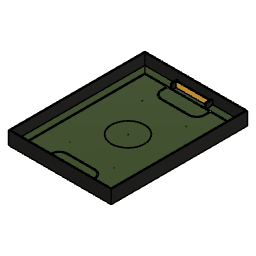
Game-field (Autodesk Fusion 360 design; units mm, degrees)
Autodesk Fusion 360 part; units mm, degrees
sketch "スケッチ1" plane through (0, 0, 0) normal (0, 1, 0) x (1, 0, 0)
  line L0 (-910, -1215) -> (910, -1215)
  line L1 (910, -1215) -> (910, 1215)
  line L2 (910, 1215) -> (-910, 1215)
  line L3 (-910, 1215) -> (-910, -1215)
  line L4 (930, 1235) -> (-930, 1235)
  line L5 (-930, 1235) -> (-930, -1235)
  line L6 (-930, -1235) -> (930, -1235)
  line L7 (930, -1235) -> (930, 1235)
extrude "押し出し1" add sketch "スケッチ1" along normal blind 20 contours L0 L1 L2 L3 | L4 L5 L6 L7
extrude "押し出し2" add sketch "スケッチ1" along normal blind 240
sketch "スケッチ2" plane through (0, 20, 0) normal (0, 1, 0) x (-1, 0, 0)
  line L0 (910, 1215) -> (-910, 1215)
  line L1 (-910, 1215) -> (-910, -1215)
  line L2 (-910, -1215) -> (910, -1215)
  line L3 (910, -1215) -> (910, 1215)
  line L4 (910, -1215) -> (-910, -1215)
  line L5 (-910, -1215) -> (-910, 1215)
  line L6 (-910, 1215) -> (910, 1215)
  line L7 (910, 1215) -> (910, -1215)
  line L8 (-810, -1115) -> (-810, 1115)
  line L9 (810, 1115) -> (810, -1115)
  line L10 (790, -1095) -> (-790, -1095)
  line L11 (-790, -1095) -> (-790, 1095)
  line L12 (-790, 1095) -> (790, 1095)
  line L13 (790, 1095) -> (790, -1095)
  circle A0 centre (400, -655) radius 5
  circle A1 centre (-400, -655) radius 5
  circle A2 centre (400, 655) radius 5
  circle A3 centre (-400, 655) radius 5
  circle A4 centre (0, 0) radius 5
  circle A5 centre (0, 0) radius 302.5
  circle A6 centre (0, 0) radius 297.5
  line L14 (-250, 845) -> (250, 845)
  line L15 (400, 995) -> (400, 1095)
  line L16 (-400, 995) -> (-400, 1095)
  arc A7 (250, 845) -> (400, 995) centre (250, 995) ccw
  arc A8 (-400, 995) -> (-250, 845) centre (-250, 995) ccw
  line L17 (-380, 995) -> (-380, 1095)
  arc A9 (-380, 995) -> (-250, 865) centre (-250, 995) ccw
  line L18 (-250, 865) -> (250, 865)
  arc A10 (250, 865) -> (380, 995) centre (250, 995) ccw
  line L19 (380, 995) -> (380, 1095)
  line L20 (300, 1169) -> (-300, 1169)
  line L21 (320, 1215) -> (320, 1095)
  line L22 (300, 1189) -> (-300, 1189)
  line L23 (-320, 1215) -> (-320, 1095)
  line L24 (-300, 1215) -> (-300, 1189)
  line L25 (-300, 1169) -> (-300, 1095)
  line L26 (300, 1215) -> (300, 1189)
  line L27 (300, 1169) -> (300, 1095)
  line L28 (320, 1115) -> (810, 1115)
  line L29 (-810, 1115) -> (-320, 1115)
  line L30 (-300, 1115) -> (300, 1115)
  line L31 (300, -1215) -> (300, -1189)
  line L32 (300, -1189) -> (-300, -1189)
  line L33 (-300, -1215) -> (-300, -1189)
  line L34 (300, -1169) -> (300, -1095)
  line L35 (-300, -1169) -> (-300, -1095)
  line L36 (300, -1169) -> (-300, -1169)
  line L37 (320, -1215) -> (320, -1095)
  line L38 (-320, -1215) -> (-320, -1095)
  line L39 (810, -1115) -> (320, -1115)
  line L40 (300, -1115) -> (-300, -1115)
  line L41 (-320, -1115) -> (-810, -1115)
  line L42 (380, -995) -> (380, -1095)
  arc A11 (380, -995) -> (250, -865) centre (250, -995) ccw
  line L43 (-250, -865) -> (250, -865)
  arc A12 (-250, -865) -> (-380, -995) centre (-250, -995) ccw
  line L44 (-380, -995) -> (-380, -1095)
  line L45 (400, -995) -> (400, -1095)
  arc A13 (400, -995) -> (250, -845) centre (250, -995) ccw
  line L46 (-250, -845) -> (250, -845)
  arc A14 (-250, -845) -> (-400, -995) centre (-250, -995) ccw
  line L47 (-400, -995) -> (-400, -1095)
  constraint coincident L0.end L1.start
  constraint coincident L2.end L3.start
  constraint coincident L12 L15.end
  constraint coincident L12 L25.end
  constraint coincident L20.start L26
  constraint coincident L20.end L24
extrude "押し出し3" add sketch "スケッチ2" along normal blind 100 contours L0 L6 L12 L20 L21 L22 L23 L24 L25 L26 L27 | L2 L4 L10 L31 L32 L33 L34 L35 L36 L37 L38
extrude "押し出し4" add sketch "スケッチ2" along normal blind 0.001 contours L9 L10 L12 L13 L21 L28 L37 L39 | L12 L25 L27 L30 | L12 L14 L15 L16 A7 A8 L17 A9 L18 A10 L19 | L8 L10 L11 L12 L23 L29 L38 L41 | L10 L42 A11 L43 A12 L44 L45 A13 L46 A14 L47 | L10 L34 L35 L40 | A0 | A1 | A2 | A3 | A4 | A5
chamfer "面取り1" distance 100 distance2 20 6 edges at (615, 20, -1215) (-615, 20, -1215) (-910, 20, 0) (615, 20, 1215) (-615, 20, 1215) (910, 20, 0) measured on face at (876.6667, 20, 371.6667) measured on face at (-876.6667, 20, 371.6667) measured on face at (-876.6667, 20, 371.6667) measured on face at (876.6667, 20, 371.6667) measured on face at (-876.6667, 20, 371.6667) measured on face at (876.6667, 20, 371.6667)
equation "d6 = 20 mm + 220 mm"
